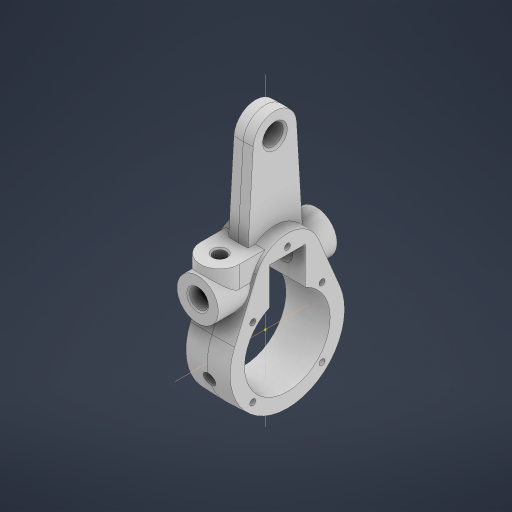
# Autodesk Inventor part: Part3
Saved by Autodesk Inventor 2023 (Build 270158000, 158)
## iProperties
Created: 2022-11-23
Part Number: Part3
Material: Generic
Document SubType Name: Modeling
Designer: iusti
Density: 1 g/cm^3
Appearance: Default
Author: iusti
Autodesk Inventor part; units mm, degrees
note: some values were not read from the file. Chosen so that the rebuilt part matches the saved one: arc direction of "Extrusion2"; direction of "Hole3"; direction of "Hole5".
ref_plane "Work Plane1" through (0, 0, 49) normal (0, 0, 1) x (1, 0, 0)
sketch "Sketch1" plane through (0, 0, 0) normal (1, 0, 0) x (0, 1, 0)
  arc A0 (16.227273, 38.738555) -> (16.227273, -38.738555) centre (0, 0) ccw
  arc A1 (53.659091, -23.058664) -> (53.659091, 23.058664) centre (44, 0) ccw
  line L0 (53.659091, 23.058664) -> (16.227273, 38.738555)
  line L1 (53.659091, -23.058664) -> (16.227273, -38.738555)
  dimension "d0" = 84
  dimension "d1" = 50
  dimension "d2" = 44
  constraints: 4 end point, 4 point on circle, 4 tangent, 2 centre point, 1 coincident, 1 horizontal alignment
  measures "d0" diameter of A0
  measures "d1" diameter of A1
  measures "d2" distance of point (0, 0) A1.centre
extrude "Extrusion1" add sketch "Sketch1" along normal mid plane 32 draft -2
sketch "Sketch2" plane through (0, 0, 0) normal (1, 0, 0) x (0, 1, 0)
  circle A0 centre (125, 0) radius 16
  arc A1 (53.443217, 22.543319) -> (53.443217, -22.543319) centre (44, 0) ccw
  line L0 (125, 0) -> (19.558732, 0)
  line L1 (125.976777, 15.970157) -> (53.092042, 20.427978)
  line L2 (125.976777, -15.970157) -> (53.092042, -20.427978)
  arc A2 (53.659091, -23.058664) -> (53.659091, 23.058664) centre (44, 0) ccw
  line L3 (53.092042, 20.427978) -> (53.092042, -20.427978)
  point P0 (0, 0)
  dimension "d5" = 32
  dimension "d6" = 125
  dimension "d9" = 3.5
  constraints: 8 end point, 3 point on circle, 1 centre point, 1 horizontal alignment, 1 tangent, 1 vertical, 1 other
  measures "d5" diameter of A0
  measures "d6" distance of point (0, 0) L0.start
  measures "d9" angle of L0 L1
sketch "Sketch2 outline for Extrusion2" plane through (0, 0, 0) normal (1, 0, 0) x (0, 1, 0)
  line L0 (125.976777, 15.970157) -> (53.092042, 20.427978)
  line L1 (53.092042, 20.427978) -> (53.092042, -20.427978)
  line L2 (53.092042, -20.427978) -> (125.976777, -15.970157)
  arc A0 (125.976777, -15.970157) -> (125.976777, 15.970157) centre (125, 0) ccw
extrude "Extrusion2" add sketch "Sketch2 outline for Extrusion2" along normal mid plane 14 draft -2
sketch "Sketch3" plane through (7, 0, 0) normal (1, 0, 0) x (0, 0, -1)
  arc A0 (-15.726167, 125.961854) -> (15.726167, 125.961854) centre (0, 125) ccw
  point P0 (0, 0)
  constraints: 1 coincident
hole "Hole1" at (7, 125, 0) direction (-1, 0, 0) diameter 15 end through all
sketch "Sketch5" plane through (0, 0, 49) normal (0, 0, 1) x (1, 0, 0)
  line L0 (0, 53.659091) -> (0, 16.227273)
  circle A0 centre (0, 43.361859) radius 15
  point P0 (0, 0)
  dimension "d29" = 30
  constraints: 1 centre point, 1 point on line
  measures "d29" diameter of A0
extrude "Extrusion4" add sketch "Sketch5" against normal blind 86
sketch "Sketch4" plane through (16, 0, 0) normal (1, 0, 0) x (0, 0, -1)
  arc A0 (-13, 28.142495) -> (13, 28.142495) centre (0, 0) ccw
  line L0 (-13, 55) -> (13, 55)
  line L1 (13, 55) -> (13, 28.142495)
  line L2 (-13, 28.142495) -> (-13, 55)
  line L3 (-13, 55) -> (13, 28.142495) construction
  line L4 (13, 55) -> (-13, 28.142495) construction
  point P0 (0, 41.571247)
  dimension "d22" = 62
  dimension "d24" = 55
  dimension "d25" = 26
  constraints: 10 end point, 2 midpoint, 2 point on circle, 1 centre point, 1 coincident, 1 horizontal, 1 parallel, 1 perpendicular, 1 vertical alignment
  measures "d22" diameter of A0
  measures "d24" distance from line of point (0, 0) L0
  measures "d25" distance between parallel lines of L1 L2
extrude "Extrusion3" cut sketch "Sketch4" against normal up to surface (32 mm away)
sketch "Sketch6" plane through (0, 43.361859, 49) normal (0, 0, 1) x (1, 0, 0)
  circle A0 centre (0, 0) radius 15 projected
  point P0 (0, -43.361859)
  point P1 (-0.001345, 15)
  constraints: 2 other
ref_plane "Work Plane2" through (-0.001345, 58.361859, 49) normal (-0.0000897, 1, 0) x (-1, -0.0000897, 0)
sketch "Sketch7" plane through (-0.001345, 58.361859, 49) normal (-0.0000897, 1, 0) x (-1, -0.0000897, 0)
  line L0 (15, 0) -> (-15, 0)
  line L1 (0, 0) -> (0, -7.948945)
  circle A0 centre (0, -16) radius 14
  line L2 (14, -16) -> (14, -34.520215)
  line L3 (14, -16) -> (32.520215, -16) construction
  line L4 (6.992592, -33.273833) -> (6.998614, -29.166963)
  ellipse E0 centre (15.999943, -49) end of major axis (15.999943, -24.558732) minor radius 0.002192 (15.999096, -26.456681) -> (15.999096, -71.543319) ccw construction
  line L5 (-14, -16) -> (-14, -34.520215)
  line L6 (-14, -16) -> (4.520215, -16) construction
  line L7 (-14, -34.520215) -> (14, -34.520215)
  line L8 (47.091032, -49) -> (-26.525387, -49)
  point P0 (0.003889, -49)
  point P1 (6.998536, -29.220211)
  point P2 (8.28839, 0)
  point P3 (-8.28839, 0)
  dimension "d33" = 28
  dimension "d34" = 90
  dimension "d35" = 90
  dimension "d42" = 33
  constraints: 13 end point, 3 perpendicular, 2 horizontal, 2 point on circle, 2 tangent, 1 centre point, 1 midpoint, 1 point on line, 1 vertical, 1 other
  measures "d33" diameter of A0
  measures "d34" angle of L2 L3
  measures "d35" angle of L5 L6
  measures "d42" distance from line of L8 A0.centre
extrude "Extrusion5" add sketch "Sketch7" along normal blind 6 and the other way blind 15
hole "Hole2" at (0, 43.361859, 49) direction (0, 0, -1) diameter 13.8 end through all
sketch "Sketch8" plane through (-0.001883, 64.361859, 49) normal (-0.0000897, 1, 0) x (1, 0.0000897, 0)
  arc A0 (-14, 16) -> (14, 16) centre (0, 16) ccw projected
  point P0 (-0.003889, 49)
  constraints: 1 coincident
hole "Hole3" at (-0.001883, 64.361859, 33) direction (0.0000897, -1, 0) diameter 8.917468 end up to surface thread size "M10x1" class "6H" standard "ISO Metric profile"
sketch "Sketch10" plane through (16, 0, 0) normal (1, 0, 0) x (0, 0, -1)
  circle A0 centre (0, 0) radius 35.5 construction
  line L0 (-25.102291, 25.102291) -> (0, 0) construction
  line L1 (60.2, 0) -> (-67.2, 0)
  line L2 (0, -78.6) -> (0, 177.6)
  point P0 (0, 60)
  point P1 (-25.102291, -25.102291)
  point P2 (25.102291, -25.102291)
  point P3 (25.102291, 25.102291)
  dimension "d66" = 71
  dimension "d67" = 45
  dimension "d68" = 60
  dimension "d71" = 360
  constraints: 2 end point, 1 coincident, 1 point on line, 8 other
  measures "d67" angle of L0 L1
  measures "d68" distance from line of L1 point (0, 60)
hole "Hole4" at (16, 60, 0) at (16, 25.102291, -25.102291) at (16, -25.102291, -25.102291) at (16, -25.102291, 25.102291) at (16, 25.102291, 25.102291) direction (-1, 0, 0) diameter 4.3 end through all
sketch "Sketch11" plane through (0, 0, 0) normal (1, 0, 0) x (0, 1, 0)
  point P0 (0, 0)
sketch "Sketch12" plane through (0, 0, 0) normal (1, 0, 0) x (0, 1, 0)
  arc A0 (16.227273, 38.738555) -> (16.227273, -38.738555) centre (0, 0) ccw
  arc A1 (28.142495, 13) -> (28.142495, -13) centre (0, 0) ccw
  line L0 (-10.8704, 40.568885) -> (0, 0) construction
  line L1 (0, -60.2) -> (0, 67.2)
  dimension "d80" = 15
  constraints: 2 end point, 1 point on circle
  measures "d80" angle of L0 L1
ref_plane "Work Plane3" through (0, -10.8704, 40.568885) normal (-0.0348995, -0.2586614, 0.9653374) x (0.9910202, -0.1337119, 0)
sketch "Sketch13" plane through (0, -10.8704, 40.568885) normal (-0.0348995, -0.2586614, 0.9653374) x (0.9910202, -0.1337119, 0)
  ellipse E0 centre (-1.453502, -0.189314) end of major axis (3.971041, -41.837535) minor radius 1.465779 (-3.623282, 5.223852) -> (-3.623282, 25.445776) ccw
  point P0 (0.002005, -0.015397)
  constraints: 2 other
hole "Hole5" at (0, -10.885398, 40.564866) direction (0.0348995, 0.2586614, -0.9653374) diameter 8.917468 end up to surface thread size "M10x1" class "6H" standard "ISO Metric profile"
chamfer "Chamfer2" distance 1 angle 45 3 edges at (-0.0019, 64.3619, 28.5413) (0, 50.2619, 49) (0, 50.2619, -37)
chamfer "Chamfer3" distance 1.5 angle 45 2 edges at (7, 125, 7.5) (-7, 125, 7.5)
body "Solid1"
